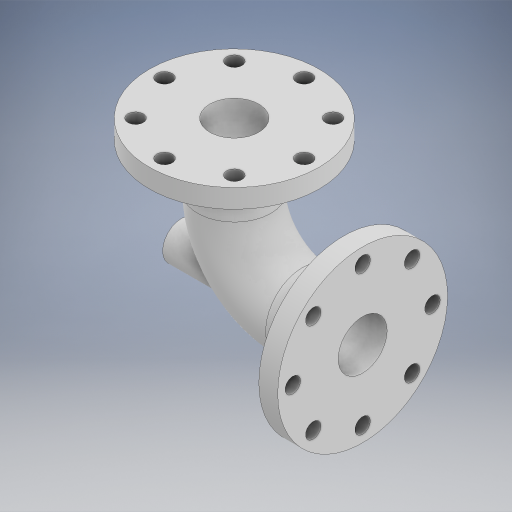
# Autodesk Inventor part: LE-2.3
Saved by Autodesk Inventor 2024 (Build 280153000, 153)
## iProperties
Created: 2024-02-01
Part Number: LE-2.3
Material: Generic
Document SubType Name: Modeling
Designer: Alex
Density: 1 g/cm^3
Appearance: Default
Author: Alex
Autodesk Inventor part; units mm, degrees
ref_plane "XZ Plane" through (0, 0, 0) normal (0, 1, 0) x (-1, 0, 0)
ref_plane "XY Plane" through (0, 0, 0) normal (0, 0, 1) x (1, 0, 0)
sketch "Sketch1" plane through (0, 0, 0) normal (0, 1, 0) x (-1, 0, 0)
  circle A0 centre (0, 0) radius 112.5
  circle A1 centre (0, 0) radius 92.5 construction
  circle A2 centre (0, 0) radius 32.5
  circle A3 centre (92.5, 0) radius 10.25
  line L0 (157.5, 0) -> (-157.5, 0) construction
  circle A4 centre (65.4074, 65.4074) radius 10.25
  circle A5 centre (0, 92.5) radius 10.25
  circle A6 centre (-65.4074, 65.4074) radius 10.25
  circle A7 centre (-92.5, 0) radius 10.25
  circle A8 centre (-65.4074, -65.4074) radius 10.25
  circle A9 centre (0, -92.5) radius 10.25
  circle A10 centre (65.4074, -65.4074) radius 10.25
  dimension "d1" = 185
  dimension "d0" = 225
  dimension "d2" = 65
  dimension "d3" = 20.5
  dimension "d6" = 360
  constraints: 10 centre point, 3 coincident, 1 horizontal alignment, 1 point on line, 19 other
  measures "d0" diameter of A0
  measures "d2" diameter of A2
  measures "d3" diameter of A3
extrude "Extrusion1" add sketch "Sketch1" against normal blind 25
sketch "Sketch2" plane through (0, 0, 0) normal (0, 0, 1) x (1, 0, 0)
  line L0 (-112.5, -25) -> (112.5, -25) projected
  line L1 (0, -25) -> (0, -85)
  line L2 (90, -175) -> (145, -175)
  arc A0 (0, -85) -> (90, -175) centre (90, -85) ccw
  line L3 (112.5, 0) -> (-112.5, 0) projected
  point P0 (0, 0)
  point P1 (0, -175)
  dimension "d13" = 145
  dimension "d14" = 90
  dimension "d27" = 175
  constraints: 4 end point, 2 point on circle, 2 point on line, 2 tangent, 1 centre point, 1 horizontal, 1 midpoint, 1 vertical
  measures "d13" distance of point (0, -175) L2.end
  measures "d14" radius of A0
  measures "d27" distance between parallel lines of L3 L2
sketch "Sketch3" plane through (0, -25, 0) normal (0, -1, 0) x (1, 0, 0)
  circle A0 centre (0, 0) radius 48.5
  circle A1 centre (0, 0) radius 32.5 projected
  dimension "d15" = 97
  constraints: 1 centre point, 1 coincident
  measures "d15" diameter of A0
sweep "Sweep1" add profiles "Sketch3" path "Sketch2" path curves L1 A0 L2
sketch "Sketch4" plane through (145, -175, 0) normal (1, 0, 0) x (0, 0, -1)
  circle A0 centre (0, 0) radius 32.5 projected
  circle A1 centre (0, 0) radius 48.5 construction
  circle A2 centre (0, 0) radius 112.5
  circle A3 centre (0, 0) radius 92.5
  line L0 (0, 0) -> (0, 112.5) construction
  circle A4 centre (0, 92.5) radius 10.25
  circle A5 centre (-65.4074, 65.4074) radius 10.25
  circle A6 centre (-92.5, 0) radius 10.25
  circle A7 centre (-65.4074, -65.4074) radius 10.25
  circle A8 centre (0, -92.5) radius 10.25
  circle A9 centre (65.4074, -65.4074) radius 10.25
  circle A10 centre (92.5, 0) radius 10.25
  circle A11 centre (65.4074, 65.4074) radius 10.25
  point P0 (0, 175)
  dimension "d18" = 225
  dimension "d19" = 185
  dimension "d20" = 20.5
  dimension "d23" = 360
  constraints: 8 centre point, 2 coincident, 2 end point, 2 vertical alignment, 1 point on line, 1 vertical, 21 other
  measures "d20" diameter of A4
extrude "Extrusion2" add sketch "Sketch4" along normal blind 25 contours A2 | A10 A3 A9 A8 A7 A6 A5 A4 A11
ref_plane "Work Plane1" through (-70, 0, 0) normal (1, 0, 0) x (0, 1, 0)
sketch "Sketch6" plane through (-70, 0, 0) normal (1, 0, 0) x (0, 1, 0)
  line L0 (0, -112.5) -> (0, 112.5) construction
  circle A0 centre (-175, 0) radius 112.5 construction
  circle A1 centre (-175, 0) radius 48.5 construction
  line L1 (0, 0) -> (-287.5, 0) construction
  circle A2 centre (-175, 0) radius 25
  dimension "d29" = 175
  dimension "d30" = 50
  constraints: 2 end point, 1 centre point, 1 horizontal, 1 horizontal alignment, 1 midpoint, 1 point on line, 1 other
  measures "d29" distance of point (0, 0) A2.centre
  measures "d30" diameter of A2
extrude "Extrusion3" add sketch "Sketch6" along normal up to next
hole "Hole1" at (-70, -175, 0) direction (1, 0, 0) diameter 20 end through all counterbore diameter 24 counterbore depth 28
body "Solid1"
